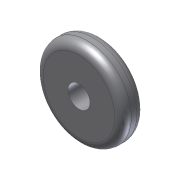
# Autodesk Inventor part: ShooterWheelConcept
Saved by Autodesk Inventor 2012 (Build 160160000, 160)
## iProperties
Created: 2012-01-18
Part Number: ShooterWheelConcept
Material: Default
Document SubType Name: Modeling
Designer: JesseK
Density: 3.13e-05 g/cm^3
Mass: 0.0453592 g
Surface Area: 905.796 cm^2
Volume: 1449.18 cm^3
Author: JesseK
Autodesk Inventor part; units mm, degrees
ref_plane "YZ Plane" through (0, 0, 0) normal (1, 0, 0) x (0, 1, 0)
ref_plane "XZ Plane" through (0, 0, 0) normal (0, 1, 0) x (-1, 0, 0)
ref_plane "XY Plane" through (0, 0, 0) normal (0, 0, 1) x (1, 0, 0)
sketch "Sketch1" plane through (0, 0, 0) normal (0, 0, 1) x (1, 0, 0)
  circle A0 centre (0, 0) radius 101.6
  dimension "d0" = 203.2
  constraints: 1 centre point, 1 coincident
  measures "d0" diameter of A0
extrude "Extrusion1" add sketch "Sketch1" along normal blind 50.8
fillet "Fillet1" radius 19.05 2 edges at (-101.6, 0, 50.8) (-101.6, 0, 0)
sketch "Sketch2" plane through (0, 0, 50.8) normal (0, 0, 1) x (1, 0, 0)
  circle A0 centre (0, 0) radius 82.55 projected
  circle A1 centre (0, 0) radius 25.4
  dimension "d4" = 50.8
  constraints: 1 centre point, 1 coincident
  measures "d4" diameter of A1
extrude "Extrusion2" cut sketch "Sketch2" against normal through all contours A1
body "Solid1"
